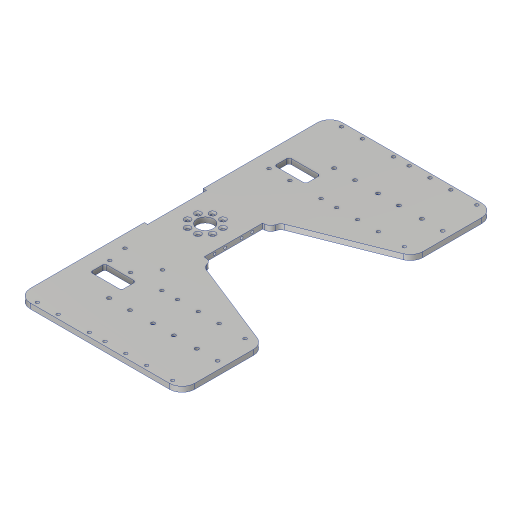
# Autodesk Inventor part: J1J2_Bottom
Saved by Autodesk Inventor 2023.2 (Build 272271000, 271)
## iProperties
Created: 2021-07-07
Part Number: J1J2_Bottom
Material: 알루미늄 6061
Document SubType Name: Modeling
Designer: user
Density: 2.7 g/cm^3
Appearance: 알루미늄 - 평지
Mass: 458.982 g
Surface Area: 798.012 cm^2
Volume: 169.993 cm^3
Author: user
Autodesk Inventor part; units mm, degrees
(part 1 of 4)
ref_plane "YZ Plane" through (0, 0, 0) normal (1, 0, 0) x (0, 1, 0)
ref_plane "XZ Plane" through (0, 0, 0) normal (0, 1, 0) x (-1, 0, 0)
ref_plane "XY Plane" through (0, 0, 0) normal (0, 0, 1) x (1, 0, 0)
sketch "스케치1" plane through (0, 0, 0) normal (0, 1, 0) x (-1, 0, 0)
  line L0 (27.1, 28) -> (-27.1, 28)
  line L1 (-27.1, 28) -> (-27.1, -28)
  line L2 (-27.1, -28) -> (27.1, -28)
  line L3 (27.1, -28) -> (27.1, 28)
  point P0 (0, 0)
  dimension "d0" = 54.2
  dimension "d1" = 56
  dimension "d2" = 27.1
  dimension "d3" = 28
  constraints: 8 end point, 2 parallel, 1 horizontal, 1 perpendicular
  measures "d0" distance of L2.end L1.end
  measures "d1" distance of L1.end L0.end
  measures "d2" distance from line of L3 point (0, 0)
  measures "d3" distance from line of L0 point (0, 0)
extrude "돌출1" add sketch "스케치1" along normal blind 5
sketch "스케치3" plane through (0, 5, 0) normal (0, 1, 0) x (1, 0, 0)
  line L0 (0, 0) -> (12.0104, 4.9749)
  line L1 (0, 0) -> (13, 0) construction
  circle A0 centre (12.0104, 4.9749) radius 1.6
  circle A1 centre (4.9749, 12.0104) radius 1.6
  circle A2 centre (-4.9749, 12.0104) radius 1.6
  circle A3 centre (-12.0104, 4.9749) radius 1.6
  circle A4 centre (-12.0104, -4.9749) radius 1.6
  circle A5 centre (-4.9749, -12.0104) radius 1.6
  circle A6 centre (4.9749, -12.0104) radius 1.6
  circle A7 centre (12.0104, -4.9749) radius 1.6
  point P0 (0, 0)
  dimension "d32" = 13
  dimension "d33" = 22.5
  dimension "d34" = 3.2
  dimension "d37" = 360
  constraints: 8 centre point, 4 end point, 1 coincident, 1 equal length, 1 horizontal, 17 other
  measures "d32" distance of L0.start L0.end
  measures "d33" angle of L1 L0
  measures "d34" diameter of A0
sketch "스케치4" plane through (0, 5, 0) normal (0, 1, 0) x (1, 0, 0)
  line L0 (27.1, 28) -> (-27.1, 28) projected
  line L1 (-27.1, -28) -> (27.1, -28) projected
  circle A0 centre (0, 0) radius 8
  line L2 (27.1, -28) -> (27.1, 28) projected
  line L3 (-27.1, 28) -> (-27.1, -28) projected
  dimension "d13" = 16
  constraints: 1 centre point, 1 coincident
  measures "d13" diameter of A0
extrude "돌출4" cut sketch "스케치4" against normal up to surface (5 mm away) contours A0
sketch "스케치5" plane through (27.1, 0, 28) normal (1, 0, 0) x (0, 0, -1)
  line L0 (0, 0) -> (56, 0) projected
  line L1 (56, 0) -> (56, 5) projected
  line L2 (0, 5) -> (56, 5) projected
  line L3 (0, 0) -> (0, 5) projected
  circle A0 centre (10, 2.5) radius 1.25
  circle A1 centre (20, 2.5) radius 1.25
  circle A2 centre (46, 2.5) radius 1.25
  circle A3 centre (36, 2.5) radius 1.25
  point P0 (28, 0)
  dimension "d16" = 2.5
  dimension "d17" = 2.5
  dimension "d18" = 2.5
  dimension "d19" = 2.5
  dimension "d20" = 2.5
  dimension "d21" = 2.5
  dimension "d22" = 2.5
  dimension "d23" = 2.5
  dimension "d24" = 10
  dimension "d25" = 20
  dimension "d26" = 20
  dimension "d27" = 10
  constraints: 4 centre point
  measures "d16" diameter of A0
  measures "d17" diameter of A1
  measures "d18" diameter of A2
  measures "d19" diameter of A3
  measures "d20" distance from line of L2 A0.centre
  measures "d21" distance from line of L2 A1.centre
  measures "d22" distance from line of L2 A2.centre
  measures "d23" distance from line of L2 A3.centre
  measures "d24" distance from line of L3 A0.centre
  measures "d25" distance from line of L3 A1.centre
  measures "d26" distance from line of L1 A3.centre
  measures "d27" distance from line of L1 A2.centre
extrude "돌출5" cut sketch "스케치5" against normal blind 8 contours A0 | A1 | A2 | A3
sketch "스케치6" plane through (-27.1, 0, -28) normal (-1, 0, 0) x (0, 0, 1)
  circle A0 centre (10, 2.5) radius 1.25 projected
  circle A1 centre (46, 2.5) radius 1.25 projected
  circle A2 centre (36, 2.5) radius 1.25 projected
  circle A3 centre (20, 2.5) radius 1.25 projected
  line L0 (56, 0) -> (0, 0) projected
  line L1 (0, 0) -> (0, 5) projected
  line L2 (56, 5) -> (0, 5) projected
  line L3 (56, 0) -> (56, 5) projected
  point P0 (28, 0)
extrude "돌출6" cut sketch "스케치6" against normal blind 8 contours A0 | A1 | A2 | A3
extrude "돌출7" cut sketch "스케치3" against normal up to surface (5 mm away)
chamfer "모따기1" distance 1.5 angle 45 8 edges at (-6.5749, 5, -12.0104) (-13.6104, 5, -4.9749) (-13.6104, 5, 4.9749) (-6.5749, 5, 12.0104) (3.3749, 5, 12.0104) (10.4104, 5, 4.9749) (10.4104, 5, -4.9749) (3.3749, 5, -12.0104)
sketch "스케치7" plane through (0, 0, 0) normal (0, -1, 0) x (1, 0, 0)
  circle A0 centre (4.9749, 12.0104) radius 1.6 projected
  circle A1 centre (12.0104, 4.9749) radius 1.6 projected
  circle A2 centre (-4.9749, 12.0104) radius 1.6 projected
  circle A3 centre (-12.0104, -4.9749) radius 1.6 projected
  circle A4 centre (4.9749, -12.0104) radius 1.6 projected
  circle A5 centre (12.0104, -4.9749) radius 1.6 projected
  circle A6 centre (-4.9749, -12.0104) radius 1.6 projected
  circle A7 centre (-12.0104, 4.9749) radius 1.6 projected
  circle A8 centre (0, 0) radius 8 projected
  line L0 (-27.1, 28) -> (27.1, 28) projected
  line L1 (-27.1, -28) -> (-27.1, 28) projected
  line L2 (27.1, -28) -> (-27.1, -28) projected
  line L3 (27.1, 28) -> (27.1, -28) projected
  line L4 (-27.1, -28) -> (-27.1, 28) projected
  line L5 (-27.1, -28) -> (156.694, -28)
  line L6 (156.694, -28) -> (156.694, -147.2716)
  line L7 (156.694, -147.2716) -> (-27.1, -147.2716)
  line L8 (-27.1, -147.2716) -> (-27.1, -28)
  line L9 (122.7787, -73) -> (-26.8765, -73)
  line L10 (-26.8765, -73) -> (-26.8765, -77)
  line L11 (-26.8765, -77) -> (122.7787, -77)
  line L12 (122.7787, -77) -> (122.7787, -73)
  line L13 (-31.8765, -68) -> (127.7787, -68)
  line L14 (127.7787, -68) -> (127.7787, -82)
  line L15 (127.7787, -82) -> (-31.8765, -82)
  line L16 (-31.8765, -82) -> (-31.8765, -68)
  point P0 (122.7787, -77)
  point P1 (-26.8765, -73)
  point P2 (-27.1, -68)
  point P3 (-27.1, -82)
  constraints: 24 end point, 4 parallel, 2 horizontal, 2 perpendicular, 4 other
extrude "돌출8" add sketch "스케치7" against normal blind 5 contours L2 L5 L6 L7 L8 L15 L14 L13
sketch "스케치9" plane through (0, 5, 0) normal (0, 1, 0) x (1, 0, 0)
  circle A0 centre (12.0104, 4.9749) radius 3.1 projected
  circle A1 centre (4.9749, -12.0104) radius 3.1 projected
  circle A2 centre (-12.0104, -4.9749) radius 3.1 projected
  circle A3 centre (-4.9749, 12.0104) radius 3.1 projected
  circle A4 centre (0, 0) radius 8 projected
  line L0 (-27.1, -28) -> (27.1, -28) projected
  line L1 (27.1, -28) -> (27.1, 28) projected
  line L2 (156.694, 28) -> (27.1, 28) projected
  line L3 (156.694, 147.2716) -> (156.694, 28) projected
  line L4 (-27.1, 147.2716) -> (156.694, 147.2716) projected
  line L5 (-27.1, 82) -> (-27.1, 147.2716) projected
  line L6 (127.7787, 82) -> (-27.1, 82) projected
  line L7 (127.7787, 68) -> (127.7787, 82) projected
  line L8 (-27.1, 68) -> (127.7787, 68) projected
  line L9 (-27.1, -28) -> (-27.1, 68) projected
  circle A5 centre (-12.0104, 4.9749) radius 3.1 projected
  circle A6 centre (-4.9749, -12.0104) radius 3.1 projected
  circle A7 centre (12.0104, -4.9749) radius 3.1 projected
  circle A8 centre (4.9749, 12.0104) radius 3.1 projected
  line L10 (57.8107, 78.5) -> (83.8107, 78.5) projected
  line L11 (127.7787, 82) -> (-27.1, 82) projected
  line L12 (83.8107, 78.5) -> (57.8107, 78.5)
  line L13 (57.8107, 78.5) -> (57.8107, 82)
  line L14 (57.8107, 82) -> (83.8107, 82)
  line L15 (83.8107, 82) -> (83.8107, 78.5)
  line L16 (70.8107, 82) -> (70.8107, 111.2)
  line L17 (70.8107, 111.2) -> (70.8107, 113.7)
  line L18 (70.8107, 96.6) -> (56.2107, 96.6)
  line L19 (56.2107, 96.6) -> (53.7107, 96.6)
  line L20 (70.8107, 96.6) -> (85.4107, 96.6)
  line L21 (85.4107, 96.6) -> (87.9107, 96.6)
  circle A9 centre (0, 0) radius 8.1
  circle A10 centre (0, 0) radius 10.1
  arc A11 (2.5, 12) -> (-2.5, 12) centre (0, 12) ccw
  arc A12 (12, -2.5) -> (12, 2.5) centre (12, 0) ccw
  arc A13 (-12, 2.5) -> (-12, -2.5) centre (-12, 0) ccw
  line L22 (2.5, 12) -> (2.5, 9.7857)
  line L23 (-2.5, 12) -> (-2.5, 9.7857)
  line L24 (-12, 2.5) -> (-9.7857, 2.5)
  line L25 (-12, -2.5) -> (-9.7857, -2.5)
  line L26 (12, 2.5) -> (9.7857, 2.5)
  line L27 (12, -2.5) -> (9.7857, -2.5)
  circle A14 centre (0, 12) radius 1.35
  circle A15 centre (12, 0) radius 1.35
  circle A16 centre (-12, 0) radius 1.35
  line L28 (58.8107, 99.1) -> (61.025, 99.1)
  line L29 (58.8107, 94.1) -> (61.025, 94.1)
  arc A17 (58.8107, 99.1) -> (58.8107, 94.1) centre (58.8107, 96.6) ccw
  circle A18 centre (58.8107, 96.6) radius 1.35
  line L30 (82.8107, 99.1) -> (80.5964, 99.1)
  circle A19 centre (82.8107, 96.6) radius 1.35
  arc A20 (82.8107, 94.1) -> (82.8107, 99.1) centre (82.8107, 96.6) ccw
  line L31 (82.8107, 94.1) -> (80.5964, 94.1)
  circle A21 centre (70.8107, 96.6) radius 8.1
  circle A22 centre (70.8107, 96.6) radius 10.1
  line L32 (68.3107, 108.6) -> (68.3107, 106.3857)
  line L33 (73.3107, 108.6) -> (73.3107, 106.3857)
  circle A23 centre (70.8107, 108.6) radius 1.35
  arc A24 (73.3107, 108.6) -> (68.3107, 108.6) centre (70.8107, 108.6) ccw
  dimension "d137" = 16.2
  dimension "d138" = 2
  dimension "d139" = 5
  dimension "d140" = 5
  dimension "d141" = 5
  dimension "d142" = 12
  dimension "d143" = 12
  dimension "d144" = 12
  dimension "d145" = 2.7
  dimension "d146" = 2.7
  dimension "d147" = 2.7
  dimension "d148" = 16.2
  dimension "d149" = 2
  dimension "d150" = 5
  dimension "d151" = 5
  dimension "d152" = 5
  dimension "d153" = 12
  dimension "d154" = 12
  dimension "d155" = 12
  dimension "d156" = 2.7
  dimension "d157" = 2.7
  dimension "d158" = 2.7
  constraints: 44 end point, 24 point on circle, 16 centre point, 11 point on line, 10 coincident, 6 tangent, 5 horizontal, 4 parallel, 4 vertical, 1 midpoint, 1 perpendicular
  measures "d137" diameter of A9
  measures "d138" radial gap between concentric circles of A9 A10
  measures "d139" diameter of A11
  measures "d140" diameter of A12
  measures "d141" diameter of A13
  measures "d142" distance of A11.centre point (0, 0)
  measures "d143" distance of A12.centre point (0, 0)
  measures "d144" distance of A13.centre point (0, 0)
  measures "d145" diameter of A14
  measures "d146" diameter of A15
  measures "d147" diameter of A16
  measures "d148" diameter of A21
  measures "d149" radial gap between concentric circles of A21 A22
  measures "d150" diameter of A24
  measures "d151" diameter of A20
  measures "d152" diameter of A17
  measures "d153" distance of A24.centre point (70.811, 96.6)
  measures "d154" distance of A20.centre point (70.811, 96.6)
  measures "d155" distance of A17.centre point (70.811, 96.6)
  measures "d156" diameter of A23
  measures "d157" diameter of A19
  measures "d158" diameter of A18
extrude "돌출9" cut sketch "스케치9" against normal blind 5 contours A18 L18 | L18 A18 | A19 L20 | L20 A19 | A23 L16 | L16 A23
sketch "스케치13" plane through (0, 5, 0) normal (0, 1, 0) x (1, 0, 0)
  line L0 (127.7787, 82) -> (-27.1, 82) projected
  line L1 (127.7787, 68) -> (127.7787, 82) projected
  line L2 (-27.1, 68) -> (127.7787, 68) projected
  line L3 (-27.1, -28) -> (-27.1, 68) projected
  line L4 (-27.1, -28) -> (27.1, -28) projected
  line L5 (27.1, -28) -> (27.1, 28) projected
  line L6 (156.694, 28) -> (27.1, 28) projected
  line L7 (156.694, 147.2716) -> (156.694, 28) projected
  line L8 (-27.1, 147.2716) -> (156.694, 147.2716) projected
  line L9 (-27.1, 82) -> (-27.1, 147.2716) projected
  circle A0 centre (12.0104, 4.9749) radius 3.1 projected
  circle A1 centre (4.9749, -12.0104) radius 3.1 projected
  circle A2 centre (-12.0104, -4.9749) radius 3.1 projected
  circle A3 centre (-4.9749, 12.0104) radius 3.1 projected
  circle A4 centre (0, 0) radius 8 projected
  circle A5 centre (-12.0104, 4.9749) radius 3.1 projected
  circle A6 centre (-4.9749, -12.0104) radius 3.1 projected
  circle A7 centre (12.0104, -4.9749) radius 3.1 projected
  circle A8 centre (4.9749, 12.0104) radius 3.1 projected
  line L10 (27.1, -28) -> (27.1, 28) projected
  line L11 (-27.1, 68) -> (127.7787, 68) projected
  line L12 (27.1, 28) -> (127.7787, 68)
  line L13 (-27.1, 82) -> (-27.1, 147.2716) projected
  line L14 (127.7787, 68) -> (-27.1, 68)
  line L15 (-27.1, 68) -> (-27.1, 147.2716)
  line L16 (-27.1, 147.2716) -> (127.7787, 147.2716)
  line L17 (127.7787, 147.2716) -> (127.7787, 68)
  line L18 (-27.1, 147.2716) -> (156.694, 147.2716) projected
  line L19 (-27.1, 147.2716) -> (127.7787, 147.2716)
  line L20 (127.7787, 147.2716) -> (127.7787, 117.4659)
  line L21 (127.7787, 117.4659) -> (-27.1, 117.4659)
  line L22 (-27.1, 117.4659) -> (-27.1, 147.2716)
  constraints: 18 end point, 4 parallel, 2 horizontal, 2 perpendicular, 1 point on line
extrude "돌출13" cut sketch "스케치13" against normal blind 500 contours L17 L8 L7 L6 L12 L1 | L21 L9 L8 L17
sketch "스케치14" plane through (0, 0, 0) normal (0, -1, 0) x (1, 0, 0)
  line L0 (-27.1, -117.4659) -> (127.7787, -117.4659) projected
  line L1 (127.7787, -117.4659) -> (127.7787, -82) projected
  line L2 (127.7787, -82) -> (-27.1, -82) projected
  line L3 (-27.1, -82) -> (-27.1, -117.4659) projected
  line L4 (127.7787, -68) -> (27.1, -28) projected
  line L5 (27.1, 28) -> (27.1, -28) projected
  line L6 (-27.1, 28) -> (27.1, 28) projected
  line L7 (-27.1, 28) -> (-27.1, -68) projected
  line L8 (-27.1, -68) -> (127.7787, -68) projected
  circle A0 centre (4.9749, 12.0104) radius 1.6 projected
  circle A1 centre (12.0104, 4.9749) radius 1.6 projected
  circle A2 centre (-4.9749, 12.0104) radius 1.6 projected
  circle A3 centre (-12.0104, -4.9749) radius 1.6 projected
  circle A4 centre (4.9749, -12.0104) radius 1.6 projected
  circle A5 centre (12.0104, -4.9749) radius 1.6 projected
  circle A6 centre (-4.9749, -12.0104) radius 1.6 projected
  circle A7 centre (-12.0104, 4.9749) radius 1.6 projected
  circle A8 centre (0, 0) radius 8 projected
  line L9 (92.0011, -83.5) -> (92.0011, -78.5) projected
  line L10 (49.6203, -83.5) -> (49.6203, -78.5) projected
  line L11 (-27.1, -68) -> (127.7787, -68) projected
  line L12 (127.7787, -82) -> (-27.1, -82) projected
  line L13 (127.7787, -68) -> (92.0011, -68)
  line L14 (92.0011, -68) -> (92.0011, -82)
  line L15 (92.0011, -82) -> (127.7787, -82)
  line L16 (127.7787, -82) -> (127.7787, -68)
  line L17 (49.6203, -82) -> (-27.1, -82)
  line L18 (-27.1, -82) -> (-27.1, -68)
  line L19 (-27.1, -68) -> (49.6203, -68)
  line L20 (49.6203, -68) -> (49.6203, -82)
  point P0 (92.0011, -82)
  constraints: 16 end point, 4 parallel, 4 point on line, 2 horizontal, 2 perpendicular
extrude "돌출14" add sketch "스케치14" against normal blind 5 contours L18 L8 L20 L10 L2 | L2 L9 L14 L8 L16
sketch "스케치15" plane through (0, 5, 0) normal (0, 1, 0) x (1, 0, 0)
  line L0 (92.0011, 82) -> (49.6203, 82) projected
  line L1 (92.0011, 68) -> (92.0011, 82) projected
  line L2 (49.6203, 68) -> (92.0011, 68) projected
  line L3 (49.6203, 82) -> (49.6203, 68) projected
  circle A0 centre (4.9749, 12.0104) radius 3.1 projected
  circle A1 centre (12.0104, -4.9749) radius 3.1 projected
  circle A2 centre (-4.9749, -12.0104) radius 3.1 projected
  circle A3 centre (-12.0104, 4.9749) radius 3.1 projected
  circle A4 centre (0, 0) radius 8 projected
  circle A5 centre (-4.9749, 12.0104) radius 3.1 projected
  circle A6 centre (-12.0104, -4.9749) radius 3.1 projected
  circle A7 centre (4.9749, -12.0104) radius 3.1 projected
  circle A8 centre (12.0104, 4.9749) radius 3.1 projected
  line L4 (-27.1, -28) -> (-27.1, 117.4659) projected
  line L5 (-27.1, -28) -> (27.1, -28) projected
  line L6 (27.1, -28) -> (27.1, 28) projected
  line L7 (27.1, 28) -> (127.7787, 68) projected
  line L8 (127.7787, 117.4659) -> (127.7787, 68) projected
  line L9 (127.7787, 117.4659) -> (-27.1, 117.4659) projected
  line L10 (127.7787, 117.4659) -> (-27.1, 117.4659) projected
  line L11 (-27.1, 117.4659) -> (15.1104, 117.4659)
  line L12 (15.1104, 117.4659) -> (15.1104, 82)
  line L13 (15.1104, 82) -> (-27.1, 82)
  line L14 (-27.1, 82) -> (-27.1, 117.4659)
  point P0 (15.1104, 117.4659)
  constraints: 8 end point, 2 parallel, 1 horizontal, 1 perpendicular
extrude "돌출15" cut sketch "스케치15" against normal blind 5 contours L4 L9 L12 L13
chamfer "모따기3" distance 2 angle 45 1 edges at (127.7787, 2.5, -68)
sketch "스케치16" plane through (0, 0, 0) normal (0, -1, 0) x (1, 0, 0)
  line L0 (49.6203, -82) -> (49.6203, -68) projected
  line L1 (49.6203, -68) -> (92.0011, -68) projected
  line L2 (92.0011, -68) -> (92.0011, -82) projected
  line L3 (92.0011, -82) -> (49.6203, -82) projected
  circle A0 centre (4.9749, 12.0104) radius 1.6 projected
  circle A1 centre (12.0104, 4.9749) radius 1.6 projected
  circle A2 centre (-4.9749, 12.0104) radius 1.6 projected
  circle A3 centre (-12.0104, -4.9749) radius 1.6 projected
  circle A4 centre (4.9749, -12.0104) radius 1.6 projected
  circle A5 centre (12.0104, -4.9749) radius 1.6 projected
  circle A6 centre (-4.9749, -12.0104) radius 1.6 projected
  circle A7 centre (-12.0104, 4.9749) radius 1.6 projected
  circle A8 centre (0, 0) radius 8 projected
  line L4 (125.92, -67.2615) -> (127.7787, -70) projected
  line L5 (125.92, -67.2615) -> (27.1, -28) projected
  line L6 (27.1, 28) -> (27.1, -28) projected
  line L7 (-27.1, 28) -> (27.1, 28) projected
  line L8 (-27.1, 28) -> (-27.1, -82) projected
  line L9 (-27.1, -82) -> (15.1104, -82) projected
  line L10 (15.1104, -82) -> (15.1104, -117.4659) projected
  line L11 (15.1104, -117.4659) -> (127.7787, -117.4659) projected
  line L12 (127.7787, -117.4659) -> (127.7787, -70) projected
  circle A9 centre (31.6, -60) radius 1 projected
  circle A10 centre (89.8107, -60) radius 1 projected
  line L13 (-24.9, -58) -> (97.8107, -58) projected
  line L14 (-24.9, -58) -> (-24.9, -62) projected
  line L15 (97.8107, -62) -> (-24.9, -62) projected
  line L16 (97.8107, -58) -> (97.8107, -62) projected
  line L17 (0, 4) -> (122.7107, 4)
  line L18 (0, 4) -> (0, 0)
  line L19 (122.7107, 0) -> (0, 0)
  line L20 (122.7107, 4) -> (122.7107, 0)
  line L21 (122.7107, 4) -> (122.7107, 0)
  line L22 (122.7107, 2) -> (114.7107, 2)
  circle A11 centre (114.7107, 2) radius 1.25
  line L23 (50.5, 0) -> (47.5, 0)
  line L24 (50.5, 4) -> (47.5, 4)
  circle A12 centre (94.7107, 2) radius 1.25
  circle A13 centre (74.7107, 2) radius 1.25
  circle A14 centre (14, 2) radius 1.25
  circle A15 centre (34, 2) radius 1.25
  line L25 (-2, 4) -> (-2, 0)
  circle A16 centre (64, 2) radius 1.25
  circle A17 centre (-10.9, -60) radius 1.6
  circle A18 centre (9.1, -60) radius 1.6
  circle A19 centre (39.1, -60) radius 1.6
  circle A20 centre (49.8107, -60) radius 1.6
  circle A21 centre (69.8107, -60) radius 1.6
  circle A22 centre (89.8107, -60) radius 1.6
  point P0 (-2, 2)
  point P1 (-24.9, -60)
  point P2 (97.8107, -60)
  dimension "d111" = 8
  dimension "d112" = 2.5
  dimension "d113" = 2.5
  dimension "d114" = 20
  dimension "d115" = 2.5
  dimension "d116" = 20
  dimension "d117" = 2.5
  dimension "d118" = 2.5
  dimension "d119" = 20
  dimension "d120" = 16
  dimension "d121" = 2.5
  dimension "d122" = 30
  dimension "d123" = 3.2
  dimension "d124" = 3.2
  dimension "d125" = 20
  dimension "d127" = 3.2
  dimension "d128" = 3.2
  dimension "d129" = 3.2
  dimension "d130" = 30
  dimension "d131" = 20
  dimension "d132" = 3.2
  dimension "d133" = 20
  dimension "d134" = 8
  dimension "d136" = 14
  constraints: 18 end point, 12 centre point, 4 midpoint, 1 coincident, 1 horizontal
  measures "d111" distance of L22.start L22.end
  measures "d112" diameter of A11
  measures "d113" diameter of A12
  measures "d114" distance of A12.centre L22.end
  measures "d115" diameter of A13
  measures "d116" distance of A13.centre A12.centre
  measures "d117" diameter of A14
  measures "d118" diameter of A15
  measures "d119" distance of A14.centre A15.centre
  measures "d120" distance of point (-2, 2) A14.centre
  measures "d121" diameter of A16
  measures "d122" distance of A15.centre A16.centre
  measures "d123" diameter of A17
  measures "d124" diameter of A18
  measures "d125" distance of A17.centre A18.centre
  measures "d127" diameter of A19
  measures "d128" diameter of A20
  measures "d129" diameter of A21
  measures "d130" distance of A19.centre A18.centre
  measures "d131" distance of A21.centre A20.centre
  measures "d132" diameter of A22
  measures "d133" distance of A21.centre A22.centre
  measures "d134" distance of point (97.811, -60) A22.centre
  measures "d136" distance of point (-24.9, -60) A17.centre
extrude "돌출16" cut sketch "스케치16" against normal blind 10 contours A10 | A17 | A18 | A19 | A20 | A21 | A22
fillet "모깎기2" radius 2 4 edges at (49.6203, 2.5, -82) (49.6203, 2.5, -68) (92.0011, 2.5, -68) (92.0011, 2.5, -82)
sketch "스케치17" plane through (0, 5, 0) normal (0, 1, 0) x (1, 0, 0)
  line L0 (127.7787, 70) -> (125.92, 67.2615) projected
  line L1 (127.7787, 117.4659) -> (127.7787, 70) projected
  line L2 (127.7787, 117.4659) -> (15.1104, 117.4659) projected
  line L3 (15.1104, 117.4659) -> (15.1104, 82) projected
  line L4 (15.1104, 82) -> (-27.1, 82) projected
  line L5 (-27.1, -28) -> (-27.1, 82) projected
  line L6 (-27.1, -28) -> (27.1, -28) projected
  line L7 (27.1, -28) -> (27.1, 28) projected
  line L8 (27.1, 28) -> (125.92, 67.2615) projected
  line L9 (90.0011, 82) -> (51.6203, 82) projected
  arc A0 (92.0011, 80) -> (90.0011, 82) centre (90.0011, 80) ccw projected
  line L10 (92.0011, 70) -> (92.0011, 80) projected
  arc A1 (90.0011, 68) -> (92.0011, 70) centre (90.0011, 70) ccw projected
  line L11 (51.6203, 68) -> (90.0011, 68) projected
  arc A2 (49.6203, 70) -> (51.6203, 68) centre (51.6203, 70) ccw projected
  line L12 (49.6203, 80) -> (49.6203, 70) projected
  arc A3 (51.6203, 82) -> (49.6203, 80) centre (51.6203, 80) ccw projected
  circle A4 centre (4.9749, 12.0104) radius 3.1 projected
  circle A5 centre (12.0104, -4.9749) radius 3.1 projected
  circle A6 centre (-4.9749, -12.0104) radius 3.1 projected
  circle A7 centre (-12.0104, 4.9749) radius 3.1 projected
  circle A8 centre (0, 0) radius 8 projected
  circle A9 centre (-4.9749, 12.0104) radius 3.1 projected
  circle A10 centre (-12.0104, -4.9749) radius 3.1 projected
  circle A11 centre (4.9749, -12.0104) radius 3.1 projected
  circle A12 centre (12.0104, 4.9749) radius 3.1 projected
  line L13 (27.1, 28) -> (125.92, 67.2615) projected
  line L14 (27.1, 28) -> (27.1, 30)
  line L15 (27.1, 30) -> (127.7787, 70)
  line L16 (-27.1, 80) -> (-27.1, 117.4659)
  line L17 (125.7787, 117.4659) -> (17.1104, 117.4659) projected
  line L18 (-27.1, 117.4659) -> (17.1104, 117.4659)
  dimension "d98" = 2
  constraints: 8 end point, 2 vertical, 1 collinear
  measures "d98" distance of L7.end L14.end
extrude "돌출17" cut sketch "스케치17" against normal blind 10 contours L0 L8 L14 L15
extrude "돌출18" add sketch "스케치17" against normal up to surface (5 mm away) contours L3 L4 L16 L18
sketch "스케치18" plane through (0, 5, 0) normal (0, 1, 0) x (1, 0, 0)
  circle A0 centre (12.0104, 4.9749) radius 3.1 projected
  circle A1 centre (4.9749, -12.0104) radius 3.1 projected
  circle A2 centre (-12.0104, -4.9749) radius 3.1 projected
  circle A3 centre (-4.9749, 12.0104) radius 3.1 projected
  circle A4 centre (0, 0) radius 8 projected
  circle A5 centre (-12.0104, 4.9749) radius 3.1 projected
  circle A6 centre (-4.9749, -12.0104) radius 3.1 projected
  circle A7 centre (12.0104, -4.9749) radius 3.1 projected
  circle A8 centre (4.9749, 12.0104) radius 3.1 projected
  line L0 (90.0011, 82) -> (51.6203, 82) projected
  arc A9 (92.0011, 80) -> (90.0011, 82) centre (90.0011, 80) ccw projected
  line L1 (92.0011, 70) -> (92.0011, 80) projected
  arc A10 (90.0011, 68) -> (92.0011, 70) centre (90.0011, 70) ccw projected
  line L2 (51.6203, 68) -> (90.0011, 68) projected
  arc A11 (49.6203, 70) -> (51.6203, 68) centre (51.6203, 70) ccw projected
  line L3 (49.6203, 80) -> (49.6203, 70) projected
  arc A12 (51.6203, 82) -> (49.6203, 80) centre (51.6203, 80) ccw projected
  line L4 (27.1, -28) -> (27.1, 30) projected
  line L5 (27.1, 30) -> (127.7787, 70) projected
  line L6 (127.7787, 117.4659) -> (127.7787, 70) projected
  line L7 (127.7787, 117.4659) -> (-27.1, 117.4659) projected
  line L8 (-27.1, 117.4659) -> (-27.1, -28) projected
  line L9 (-27.1, -28) -> (27.1, -28) projected
  line L10 (92.0011, 70) -> (92.0011, 80) projected
  line L11 (92.0011, 75) -> (-27.1, 75)
  line L12 (-27.1, 117.4659) -> (-27.1, -28) projected
  line L13 (-15, 68) -> (15, 68)
  line L14 (15, 68) -> (15, 82)
  line L15 (15, 82) -> (-15, 82)
  line L16 (-15, 82) -> (-15, 68)
  line L17 (-15, 68) -> (15, 82) construction
  line L18 (15, 68) -> (-15, 82) construction
  point P0 (0, 75)
  dimension "d103" = 30
  constraints: 14 end point, 3 midpoint, 3 point on line, 2 parallel, 2 perpendicular, 1 horizontal
  measures "d103" distance of L15.end L14.end
extrude "돌출19" cut sketch "스케치18" against normal blind 10 contours L14 L13 L16 L11 | L11 L16 L15 L14
sketch "스케치19" plane through (0, 5, 0) normal (0, 1, 0) x (1, 0, 0)
  line L0 (-15, 82) -> (15, 82) projected
  line L1 (15, 82) -> (15, 68) projected
  line L2 (15, 68) -> (-15, 68) projected
  line L3 (-15, 68) -> (-15, 82) projected
  circle A0 centre (12.0104, 4.9749) radius 3.1 projected
  circle A1 centre (4.9749, -12.0104) radius 3.1 projected
  circle A2 centre (-12.0104, -4.9749) radius 3.1 projected
  circle A3 centre (-4.9749, 12.0104) radius 3.1 projected
  circle A4 centre (0, 0) radius 8 projected
  circle A5 centre (-12.0104, 4.9749) radius 3.1 projected
  circle A6 centre (-4.9749, -12.0104) radius 3.1 projected
  circle A7 centre (12.0104, -4.9749) radius 3.1 projected
  circle A8 centre (4.9749, 12.0104) radius 3.1 projected
  line L4 (90.0011, 82) -> (51.6203, 82) projected
  arc A9 (92.0011, 80) -> (90.0011, 82) centre (90.0011, 80) ccw projected
  line L5 (92.0011, 70) -> (92.0011, 80) projected
  arc A10 (90.0011, 68) -> (92.0011, 70) centre (90.0011, 70) ccw projected
  line L6 (51.6203, 68) -> (90.0011, 68) projected
  arc A11 (49.6203, 70) -> (51.6203, 68) centre (51.6203, 70) ccw projected
  line L7 (49.6203, 80) -> (49.6203, 70) projected
  arc A12 (51.6203, 82) -> (49.6203, 80) centre (51.6203, 80) ccw projected
  line L8 (27.1, -28) -> (27.1, 30) projected
  line L9 (27.1, 30) -> (127.7787, 70) projected
  line L10 (127.7787, 117.4659) -> (127.7787, 70) projected
  line L11 (127.7787, 117.4659) -> (-27.1, 117.4659) projected
  line L12 (-27.1, 117.4659) -> (-27.1, -28) projected
  line L13 (-27.1, -28) -> (27.1, -28) projected
  line L14 (-27.1, -28) -> (-27.1, 117.4659) projected
  line L15 (-27.1, 97.4659) -> (12.9, 117.4659)
  line L16 (-27.1, 117.4659) -> (125.7787, 117.4659) projected
  dimension "d106" = 20
  dimension "d107" = 40
  constraints: 2 end point, 2 point on line
  measures "d106" distance from line of L15.start L16
  measures "d107" distance from line of L12 L15.end
extrude "돌출20" cut sketch "스케치19" against normal blind 10 contours L12 L11 L15
fillet "모깎기3" radius 2 9 edges at (15, 2.5, -68) (15, 2.5, -82) (-15, 2.5, -68) (-15, 2.5, -82) (-27.1, 2.5, -97.4659) (12.9, 2.5, -117.4659) (127.7787, 2.5, -117.4659) (127.7787, 2.5, -70) (27.1, 2.5, -30)
sketch "스케치20" plane through (0, 5, 0) normal (0, 1, 0) x (1, 0, 0)
  arc A0 (126.5171, 69.4988) -> (127.7787, 71.3575) centre (125.7787, 71.3575) ccw projected
  line L0 (127.7787, 115.4659) -> (127.7787, 71.3575) projected
  arc A1 (127.7787, 115.4659) -> (125.7787, 117.4659) centre (125.7787, 115.4659) ccw projected
  line L1 (125.7787, 117.4659) -> (13.3721, 117.4659) projected
  arc A2 (13.3721, 117.4659) -> (12.4777, 117.2547) centre (13.3721, 115.4659) ccw projected
  line L2 (12.4777, 117.2547) -> (-25.9944, 98.0187) projected
  arc A3 (-25.9944, 98.0187) -> (-27.1, 96.2298) centre (-25.1, 96.2298) ccw projected
  line L3 (-27.1, 96.2298) -> (-27.1, -28) projected
  line L4 (-27.1, -28) -> (27.1, -28) projected
  line L5 (27.1, -28) -> (27.1, 28.6425) projected
  arc A4 (28.3615, 30.5012) -> (27.1, 28.6425) centre (29.1, 28.6425) ccw projected
  line L6 (28.3615, 30.5012) -> (126.5171, 69.4988) projected
  line L7 (15, 80) -> (15, 70) projected
  arc A5 (13, 68) -> (15, 70) centre (13, 70) ccw projected
  line L8 (13, 68) -> (-13, 68) projected
  arc A6 (-15, 70) -> (-13, 68) centre (-13, 70) ccw projected
  line L9 (-15, 70) -> (-15, 80) projected
  arc A7 (-13, 82) -> (-15, 80) centre (-13, 80) ccw projected
  line L10 (-13, 82) -> (13, 82) projected
  arc A8 (15, 80) -> (13, 82) centre (13, 80) ccw projected
  arc A9 (92.0011, 80) -> (90.0011, 82) centre (90.0011, 80) ccw projected
  line L11 (92.0011, 70) -> (92.0011, 80) projected
  arc A10 (90.0011, 68) -> (92.0011, 70) centre (90.0011, 70) ccw projected
  line L12 (51.6203, 68) -> (90.0011, 68) projected
  arc A11 (49.6203, 70) -> (51.6203, 68) centre (51.6203, 70) ccw projected
  line L13 (49.6203, 80) -> (49.6203, 70) projected
  arc A12 (51.6203, 82) -> (49.6203, 80) centre (51.6203, 80) ccw projected
  line L14 (90.0011, 82) -> (51.6203, 82) projected
  circle A13 centre (82.8107, 96.6) radius 1.35 projected
  circle A14 centre (58.8107, 96.6) radius 1.35 projected
  circle A15 centre (70.8107, 108.6) radius 1.35 projected
  circle A16 centre (4.9749, 12.0104) radius 3.1 projected
  circle A17 centre (12.0104, -4.9749) radius 3.1 projected
  circle A18 centre (-4.9749, -12.0104) radius 3.1 projected
  circle A19 centre (-12.0104, 4.9749) radius 3.1 projected
  circle A20 centre (0, 0) radius 8 projected
  circle A21 centre (-4.9749, 12.0104) radius 3.1 projected
  circle A22 centre (-12.0104, -4.9749) radius 3.1 projected
  circle A23 centre (4.9749, -12.0104) radius 3.1 projected
  circle A24 centre (12.0104, 4.9749) radius 3.1 projected
  circle A25 centre (89.8107, 60) radius 1.6 projected
  circle A26 centre (9.1, 60) radius 1.6 projected
  circle A27 centre (39.1, 60) radius 1.6 projected
  circle A28 centre (69.8107, 60) radius 1.6 projected
  circle A29 centre (-10.9, 60) radius 1.6 projected
  circle A30 centre (49.8107, 60) radius 1.6 projected
  line L15 (127.7787, 115.4659) -> (127.7787, 117.4659)
  line L16 (127.7787, 117.4659) -> (127.7787, 133.9669)
  line L17 (127.7787, 133.9669) -> (13, 133.9669)
  line L18 (13, 133.9669) -> (-27.1, 113.9169)
  line L19 (-27.1, -28) -> (-27.1, 96.2298) projected
  line L20 (-27.1, 96.2298) -> (-27.1, 113.9169)
  dimension "d159" = 16.501
  constraints: 10 end point, 2 vertical, 1 collinear, 1 parallel, 1 perpendicular, 1 tangent
  measures "d159" distance of L15.end L16.end
extrude "돌출21" add sketch "스케치20" against normal blind 5 contours A1 L1 A2 L2 A3 L20 L18 L17 L16 L15
sketch "스케치21" plane through (0, 5, 0) normal (0, 1, 0) x (1, 0, 0)
  arc A0 (126.5171, 69.4988) -> (127.7787, 71.3575) centre (125.7787, 71.3575) ccw projected
  line L0 (127.7787, 133.9669) -> (127.7787, 71.3575) projected
  line L1 (127.7787, 133.9669) -> (13, 133.9669) projected
  line L2 (13, 133.9669) -> (-27.1, 113.9169) projected
  line L3 (-27.1, 113.9169) -> (-27.1, -28) projected
  line L4 (-27.1, -28) -> (27.1, -28) projected
  line L5 (27.1, -28) -> (27.1, 28.6425) projected
  arc A1 (28.3615, 30.5012) -> (27.1, 28.6425) centre (29.1, 28.6425) ccw projected
  line L6 (28.3615, 30.5012) -> (126.5171, 69.4988) projected
  line L7 (15, 80) -> (15, 70) projected
  arc A2 (13, 68) -> (15, 70) centre (13, 70) ccw projected
  line L8 (13, 68) -> (-13, 68) projected
  arc A3 (-15, 70) -> (-13, 68) centre (-13, 70) ccw projected
  line L9 (-15, 70) -> (-15, 80) projected
  arc A4 (-13, 82) -> (-15, 80) centre (-13, 80) ccw projected
  line L10 (-13, 82) -> (13, 82) projected
  arc A5 (15, 80) -> (13, 82) centre (13, 80) ccw projected
  arc A6 (92.0011, 80) -> (90.0011, 82) centre (90.0011, 80) ccw projected
  line L11 (92.0011, 70) -> (92.0011, 80) projected
  arc A7 (90.0011, 68) -> (92.0011, 70) centre (90.0011, 70) ccw projected
  line L12 (51.6203, 68) -> (90.0011, 68) projected
  arc A8 (49.6203, 70) -> (51.6203, 68) centre (51.6203, 70) ccw projected
  line L13 (49.6203, 80) -> (49.6203, 70) projected
  arc A9 (51.6203, 82) -> (49.6203, 80) centre (51.6203, 80) ccw projected
  line L14 (90.0011, 82) -> (51.6203, 82) projected
  circle A10 centre (82.8107, 96.6) radius 1.35 projected
  circle A11 centre (58.8107, 96.6) radius 1.35 projected
  circle A12 centre (70.8107, 108.6) radius 1.35 projected
  circle A13 centre (4.9749, 12.0104) radius 3.1 projected
  circle A14 centre (12.0104, -4.9749) radius 3.1 projected
  circle A15 centre (-4.9749, -12.0104) radius 3.1 projected
  circle A16 centre (-12.0104, 4.9749) radius 3.1 projected
  circle A17 centre (0, 0) radius 8 projected
  circle A18 centre (-4.9749, 12.0104) radius 3.1 projected
  circle A19 centre (-12.0104, -4.9749) radius 3.1 projected
  circle A20 centre (4.9749, -12.0104) radius 3.1 projected
  circle A21 centre (12.0104, 4.9749) radius 3.1 projected
  circle A22 centre (89.8107, 60) radius 1.6 projected
  circle A23 centre (9.1, 60) radius 1.6 projected
  circle A24 centre (39.1, 60) radius 1.6 projected
  circle A25 centre (69.8107, 60) radius 1.6 projected
  circle A26 centre (-10.9, 60) radius 1.6 projected
  circle A27 centre (49.8107, 60) radius 1.6 projected
  arc A28 (126.5171, 85.9998) -> (127.7787, 87.8585) centre (125.7787, 87.8585) ccw
  line L15 (127.7787, 150.4679) -> (127.7787, 87.8585)
  line L16 (127.7787, 150.4679) -> (13, 150.4679)
  line L17 (13, 150.4679) -> (-27.1, 130.4179)
  line L18 (-27.1, 130.4179) -> (-27.1, -11.499)
  line L19 (-27.1, -11.499) -> (27.1, -11.499)
  line L20 (27.1, -11.499) -> (27.1, 45.1435)
  arc A29 (28.3615, 47.0022) -> (27.1, 45.1435) centre (29.1, 45.1435) ccw
  line L21 (28.3615, 47.0022) -> (126.5171, 85.9998)
  line L22 (15, 96.501) -> (15, 86.501)
  arc A30 (13, 84.501) -> (15, 86.501) centre (13, 86.501) ccw
  line L23 (13, 84.501) -> (-13, 84.501)
  arc A31 (-15, 86.501) -> (-13, 84.501) centre (-13, 86.501) ccw
  line L24 (-15, 86.501) -> (-15, 96.501)
  arc A32 (-13, 98.501) -> (-15, 96.501) centre (-13, 96.501) ccw
  line L25 (-13, 98.501) -> (13, 98.501)
  arc A33 (15, 96.501) -> (13, 98.501) centre (13, 96.501) ccw
  arc A34 (92.0011, 96.501) -> (90.0011, 98.501) centre (90.0011, 96.501) ccw
  line L26 (92.0011, 86.501) -> (92.0011, 96.501)
  arc A35 (90.0011, 84.501) -> (92.0011, 86.501) centre (90.0011, 86.501) ccw
  line L27 (51.6203, 84.501) -> (90.0011, 84.501)
  arc A36 (49.6203, 86.501) -> (51.6203, 84.501) centre (51.6203, 86.501) ccw
  line L28 (49.6203, 96.501) -> (49.6203, 86.501)
  arc A37 (51.6203, 98.501) -> (49.6203, 96.501) centre (51.6203, 96.501) ccw
  line L29 (90.0011, 98.501) -> (51.6203, 98.501)
  circle A38 centre (82.8107, 113.101) radius 1.35
  circle A39 centre (58.8107, 113.101) radius 1.35
  circle A40 centre (70.8107, 125.101) radius 1.35
  circle A41 centre (112.9107, 103.101) radius 1.75
  circle A42 centre (28.7107, 103.101) radius 1.75
  circle A43 centre (112.9107, 123.101) radius 1.75
  circle A44 centre (28.7107, 123.101) radius 1.75
  circle A45 centre (4.9749, 28.5114) radius 3.1
  circle A46 centre (12.0104, 11.5261) radius 3.1
  circle A47 centre (-4.9749, 4.4906) radius 3.1
  circle A48 centre (-12.0104, 21.4759) radius 3.1
  circle A49 centre (0, 16.501) radius 8
  circle A50 centre (-4.9749, 28.5114) radius 3.1
  circle A51 centre (-12.0104, 11.5261) radius 3.1
  circle A52 centre (4.9749, 4.4906) radius 3.1
  circle A53 centre (12.0104, 21.4759) radius 3.1
  circle A54 centre (89.8107, 76.501) radius 1.6
  circle A55 centre (9.1, 76.501) radius 1.6
  circle A56 centre (39.1, 76.501) radius 1.6
  circle A57 centre (69.8107, 76.501) radius 1.6
  circle A58 centre (-10.9, 76.501) radius 1.6
  circle A59 centre (49.8107, 76.501) radius 1.6
  circle A60 centre (-10.9, 60) radius 1.6 projected
  line L30 (-10.9, 60) -> (-10.9, 76.501)
  point P0 (0, 16.501)
  point P1 (81.2123, 68)
  point P2 (92.0011, 72.2864)
  point P3 (127.7787, 87.8585)
  dimension "d162" = 16.501
  constraints: 32 centre point, 32 end point, 20 point on circle, 1 vertical
  measures "d162" distance of L30.start L30.end
extrude "돌출22" add sketch "스케치21" against normal blind 5 contours L21 L12 A8 L13 A59 A9 L14 A6 L11 | L13 A59 | L7 A2 L8 A3 L9 A4 L10 A5 | A10 | A11 | A12 | A23 | A24 | A26 | A27 picked at (50.6624, 76.7486)
extrude "돌출23" cut sketch "스케치21" against normal blind 5 contours L6 A1 L20 A29 L21 L12 A7 L11 A28 L0 A0 | A59 L13 | L13 A59 | A10 | A11 | L22 A30 L23 A31 L24 A32 L25 A33 | L26 A35 L27 A36 L28 A37 L29 A34 | A38 | A39 | A40 | A41 | A42 | A43 | A44 | A56
sketch "스케치22" plane through (0, 5, 0) normal (0, 1, 0) x (1, 0, 0)
  line L0 (28.3615, 47.0022) -> (126.5171, 85.9998) projected
  arc A0 (126.5171, 85.9998) -> (127.7787, 87.8585) centre (125.7787, 87.8585) ccw projected
  line L1 (127.7787, 133.9669) -> (127.7787, 87.8585) projected
  line L2 (127.7787, 133.9669) -> (13, 133.9669) projected
  line L3 (13, 133.9669) -> (-27.1, 113.9169) projected
  line L4 (-27.1, 113.9169) -> (-27.1, -28) projected
  line L5 (-27.1, -28) -> (27.1, -28) projected
  line L6 (27.1, -28) -> (27.1, 45.1435) projected
  arc A1 (28.3615, 47.0022) -> (27.1, 45.1435) centre (29.1, 45.1435) ccw projected
  arc A2 (15, 96.501) -> (13, 98.501) centre (13, 96.501) ccw projected
  line L7 (15, 96.501) -> (15, 86.501) projected
  arc A3 (13, 84.501) -> (15, 86.501) centre (13, 86.501) ccw projected
  line L8 (13, 84.501) -> (-13, 84.501) projected
  arc A4 (-15, 86.501) -> (-13, 84.501) centre (-13, 86.501) ccw projected
  line L9 (-15, 86.501) -> (-15, 96.501) projected
  arc A5 (-13, 98.501) -> (-15, 96.501) centre (-13, 96.501) ccw projected
  line L10 (-13, 98.501) -> (13, 98.501) projected
  circle A6 centre (58.8107, 113.101) radius 1.35 projected
  circle A7 centre (112.9107, 103.101) radius 1.75 projected
  circle A8 centre (28.7107, 123.101) radius 1.75 projected
  circle A9 centre (82.8107, 113.101) radius 1.35 projected
  line L11 (51.6203, 98.501) -> (90.0011, 98.501) projected
  arc A10 (92.0011, 96.501) -> (90.0011, 98.501) centre (90.0011, 96.501) ccw projected
  line L12 (92.0011, 96.501) -> (92.0011, 86.501) projected
  arc A11 (90.0011, 84.501) -> (92.0011, 86.501) centre (90.0011, 86.501) ccw projected
  line L13 (90.0011, 84.501) -> (51.6203, 84.501) projected
  arc A12 (49.6203, 86.501) -> (51.6203, 84.501) centre (51.6203, 86.501) ccw projected
  line L14 (49.6203, 86.501) -> (49.6203, 96.501) projected
  arc A13 (51.6203, 98.501) -> (49.6203, 96.501) centre (51.6203, 96.501) ccw projected
  circle A14 centre (39.1, 76.501) radius 1.6 projected
  circle A15 centre (70.8107, 125.101) radius 1.35 projected
  circle A16 centre (112.9107, 123.101) radius 1.75 projected
  circle A17 centre (28.7107, 103.101) radius 1.75 projected
  circle A18 centre (49.8107, 76.501) radius 1.6 projected
  circle A19 centre (9.1, 76.501) radius 1.6 projected
  circle A20 centre (-10.9, 76.501) radius 1.6 projected
  circle A21 centre (69.8107, 76.501) radius 1.6 projected
  circle A22 centre (89.8107, 76.501) radius 1.6 projected
  circle A23 centre (12.0104, 4.9749) radius 3.1 projected
  circle A24 centre (4.9749, -12.0104) radius 3.1 projected
  circle A25 centre (-12.0104, -4.9749) radius 3.1 projected
  circle A26 centre (-4.9749, 12.0104) radius 3.1 projected
  circle A27 centre (0, 0) radius 8 projected
  circle A28 centre (-12.0104, 4.9749) radius 3.1 projected
  circle A29 centre (-4.9749, -12.0104) radius 3.1 projected
  circle A30 centre (12.0104, -4.9749) radius 3.1 projected
  circle A31 centre (4.9749, 12.0104) radius 3.1 projected
  line L15 (28.3615, 44.0022) -> (126.5171, 82.9998)
  arc A32 (126.5171, 82.9998) -> (127.7787, 84.8585) centre (125.7787, 84.8585) ccw
  line L16 (127.7787, 130.9669) -> (127.7787, 84.8585)
  line L17 (127.7787, 130.9669) -> (13, 130.9669)
  line L18 (13, 130.9669) -> (-27.1, 110.9169)
  line L19 (-27.1, 110.9169) -> (-27.1, -31)
  line L20 (-27.1, -31) -> (27.1, -31)
  line L21 (27.1, -31) -> (27.1, 42.1435)
  arc A33 (28.3615, 44.0022) -> (27.1, 42.1435) centre (29.1, 42.1435) ccw
  arc A34 (15, 93.501) -> (13, 95.501) centre (13, 93.501) ccw
  line L22 (15, 93.501) -> (15, 83.501)
  arc A35 (13, 81.501) -> (15, 83.501) centre (13, 83.501) ccw
  line L23 (13, 81.501) -> (-13, 81.501)
  arc A36 (-15, 83.501) -> (-13, 81.501) centre (-13, 83.501) ccw
  line L24 (-15, 83.501) -> (-15, 93.501)
  arc A37 (-13, 95.501) -> (-15, 93.501) centre (-13, 93.501) ccw
  line L25 (-13, 95.501) -> (13, 95.501)
  circle A38 centre (58.8107, 110.101) radius 1.35
  circle A39 centre (112.9107, 100.101) radius 1.75
  circle A40 centre (28.7107, 120.101) radius 1.75
  circle A41 centre (82.8107, 110.101) radius 1.35
  line L26 (51.6203, 95.501) -> (90.0011, 95.501)
  arc A42 (92.0011, 93.501) -> (90.0011, 95.501) centre (90.0011, 93.501) ccw
  line L27 (92.0011, 93.501) -> (92.0011, 83.501)
  arc A43 (90.0011, 81.501) -> (92.0011, 83.501) centre (90.0011, 83.501) ccw
  line L28 (90.0011, 81.501) -> (51.6203, 81.501)
  arc A44 (49.6203, 83.501) -> (51.6203, 81.501) centre (51.6203, 83.501) ccw
  line L29 (49.6203, 83.501) -> (49.6203, 93.501)
  arc A45 (51.6203, 95.501) -> (49.6203, 93.501) centre (51.6203, 93.501) ccw
  circle A46 centre (39.1, 73.501) radius 1.6
  circle A47 centre (70.8107, 122.101) radius 1.35
  circle A48 centre (112.9107, 120.101) radius 1.75
  circle A49 centre (28.7107, 100.101) radius 1.75
  circle A50 centre (49.8107, 73.501) radius 1.6
  circle A51 centre (9.1, 73.501) radius 1.6
  circle A52 centre (-10.9, 73.501) radius 1.6
  circle A53 centre (69.8107, 73.501) radius 1.6
  circle A54 centre (89.8107, 73.501) radius 1.6
  circle A55 centre (12.0104, 1.9749) radius 3.1
  circle A56 centre (4.9749, -15.0104) radius 3.1
  circle A57 centre (-12.0104, -7.9749) radius 3.1
  circle A58 centre (-4.9749, 9.0104) radius 3.1
  circle A59 centre (0, -3) radius 8
  circle A60 centre (-12.0104, 1.9749) radius 3.1
  circle A61 centre (-4.9749, -15.0104) radius 3.1
  circle A62 centre (12.0104, -7.9749) radius 3.1
  circle A63 centre (4.9749, 9.0104) radius 3.1
  line L30 (-13, 86.501) -> (-13, 83.501)
  point P0 (-15, 93.501)
  point P1 (49.6203, 86.501)
  point P2 (-15, 86.501)
  dimension "d167" = 3
  constraints: 32 centre point, 32 end point, 20 point on circle, 1 vertical
  measures "d167" distance of L30.start L30.end
extrude "돌출24" add sketch "스케치22" against normal blind 5 contours L7 A34 L25 A37 L9 A5 L10 A2 | L11 A10 L12 A42 L26 A45 L14 A13
extrude "돌출25" cut sketch "스케치22" against normal blind 5 contours L22 A35 L23 A36 L24 A4 L8 A3 | A12 L13 A11 L27 A43 L28 A44 L29
sketch "스케치23" plane through (0, 5, 0) normal (0, 1, 0) x (1, 0, 0)
  circle A0 centre (4.9749, 12.0104) radius 3.1 projected
  circle A1 centre (12.0104, -4.9749) radius 3.1 projected
  circle A2 centre (-4.9749, -12.0104) radius 3.1 projected
  circle A3 centre (-12.0104, 4.9749) radius 3.1 projected
  circle A4 centre (0, 0) radius 8 projected
  circle A5 centre (-4.9749, 12.0104) radius 3.1 projected
  circle A6 centre (-12.0104, -4.9749) radius 3.1 projected
  circle A7 centre (4.9749, -12.0104) radius 3.1 projected
  circle A8 centre (12.0104, 4.9749) radius 3.1 projected
  circle A9 centre (89.8107, 76.501) radius 1.6 projected
  circle A10 centre (69.8107, 76.501) radius 1.6 projected
  circle A11 centre (-10.9, 76.501) radius 1.6 projected
  circle A12 centre (9.1, 76.501) radius 1.6 projected
  circle A13 centre (49.8107, 76.501) radius 1.6 projected
  circle A14 centre (28.7107, 103.101) radius 1.75 projected
  circle A15 centre (112.9107, 123.101) radius 1.75 projected
  circle A16 centre (70.8107, 125.101) radius 1.35 projected
  circle A17 centre (39.1, 76.501) radius 1.6 projected
  circle A18 centre (82.8107, 113.101) radius 1.35 projected
  circle A19 centre (28.7107, 123.101) radius 1.75 projected
  circle A20 centre (112.9107, 103.101) radius 1.75 projected
  circle A21 centre (58.8107, 113.101) radius 1.35 projected
  line L0 (15, 93.501) -> (15, 83.501) projected
  arc A22 (13, 81.501) -> (15, 83.501) centre (13, 83.501) ccw projected
  line L1 (13, 81.501) -> (-13, 81.501) projected
  arc A23 (-15, 83.501) -> (-13, 81.501) centre (-13, 83.501) ccw projected
  line L2 (-15, 83.501) -> (-15, 93.501) projected
  arc A24 (-13, 95.501) -> (-15, 93.501) centre (-13, 93.501) ccw projected
  line L3 (-13, 95.501) -> (13, 95.501) projected
  arc A25 (15, 93.501) -> (13, 95.501) centre (13, 93.501) ccw projected
  line L4 (28.3615, 47.0022) -> (126.5171, 85.9998) projected
  arc A26 (126.5171, 85.9998) -> (127.7787, 87.8585) centre (125.7787, 87.8585) ccw projected
  line L5 (127.7787, 133.9669) -> (127.7787, 87.8585) projected
  line L6 (127.7787, 133.9669) -> (13, 133.9669) projected
  line L7 (13, 133.9669) -> (-27.1, 113.9169) projected
  line L8 (-27.1, 113.9169) -> (-27.1, -28) projected
  line L9 (-27.1, -28) -> (27.1, -28) projected
  line L10 (27.1, -28) -> (27.1, 45.1435) projected
  arc A27 (28.3615, 47.0022) -> (27.1, 45.1435) centre (29.1, 45.1435) ccw projected
  line L11 (49.6203, 83.501) -> (49.6203, 93.501) projected
  arc A28 (51.6203, 95.501) -> (49.6203, 93.501) centre (51.6203, 93.501) ccw projected
  line L12 (51.6203, 95.501) -> (90.0011, 95.501) projected
  arc A29 (92.0011, 93.501) -> (90.0011, 95.501) centre (90.0011, 93.501) ccw projected
  line L13 (92.0011, 93.501) -> (92.0011, 83.501) projected
  arc A30 (90.0011, 81.501) -> (92.0011, 83.501) centre (90.0011, 83.501) ccw projected
  line L14 (90.0011, 81.501) -> (51.6203, 81.501) projected
  arc A31 (49.6203, 83.501) -> (51.6203, 81.501) centre (51.6203, 83.501) ccw projected
  circle A32 centre (4.9749, 5.0104) radius 3.1
  circle A33 centre (12.0104, -11.9749) radius 3.1
  circle A34 centre (-4.9749, -19.0104) radius 3.1
  circle A35 centre (-12.0104, -2.0251) radius 3.1
  circle A36 centre (0, -7) radius 8
  circle A37 centre (-4.9749, 5.0104) radius 3.1
  circle A38 centre (-12.0104, -11.9749) radius 3.1
  circle A39 centre (4.9749, -19.0104) radius 3.1
  circle A40 centre (12.0104, -2.0251) radius 3.1
  circle A41 centre (89.8107, 69.501) radius 1.6
  circle A42 centre (69.8107, 69.501) radius 1.6
  circle A43 centre (-10.9, 69.501) radius 1.6
  circle A44 centre (9.1, 69.501) radius 1.6
  circle A45 centre (49.8107, 69.501) radius 1.6
  circle A46 centre (28.7107, 96.101) radius 1.75
  circle A47 centre (112.9107, 116.101) radius 1.75
  circle A48 centre (70.8107, 118.101) radius 1.35
  circle A49 centre (39.1, 69.501) radius 1.6
  circle A50 centre (82.8107, 106.101) radius 1.35
  circle A51 centre (28.7107, 116.101) radius 1.75
  circle A52 centre (112.9107, 96.101) radius 1.75
  circle A53 centre (58.8107, 106.101) radius 1.35
  line L15 (15, 86.501) -> (15, 76.501)
  arc A54 (13, 74.501) -> (15, 76.501) centre (13, 76.501) ccw
  line L16 (13, 74.501) -> (-13, 74.501)
  arc A55 (-15, 76.501) -> (-13, 74.501) centre (-13, 76.501) ccw
  line L17 (-15, 76.501) -> (-15, 86.501)
  arc A56 (-13, 88.501) -> (-15, 86.501) centre (-13, 86.501) ccw
  line L18 (-13, 88.501) -> (13, 88.501)
  arc A57 (15, 86.501) -> (13, 88.501) centre (13, 86.501) ccw
  line L19 (28.3615, 40.0022) -> (126.5171, 78.9998)
  arc A58 (126.5171, 78.9998) -> (127.7787, 80.8585) centre (125.7787, 80.8585) ccw
  line L20 (127.7787, 126.9669) -> (127.7787, 80.8585)
  line L21 (127.7787, 126.9669) -> (13, 126.9669)
  line L22 (13, 126.9669) -> (-27.1, 106.9169)
  line L23 (-27.1, 106.9169) -> (-27.1, -35)
  line L24 (-27.1, -35) -> (27.1, -35)
  line L25 (27.1, -35) -> (27.1, 38.1435)
  arc A59 (28.3615, 40.0022) -> (27.1, 38.1435) centre (29.1, 38.1435) ccw
  line L26 (49.6203, 76.501) -> (49.6203, 86.501)
  arc A60 (51.6203, 88.501) -> (49.6203, 86.501) centre (51.6203, 86.501) ccw
  line L27 (51.6203, 88.501) -> (90.0011, 88.501)
  arc A61 (92.0011, 86.501) -> (90.0011, 88.501) centre (90.0011, 86.501) ccw
  line L28 (92.0011, 86.501) -> (92.0011, 76.501)
  arc A62 (90.0011, 74.501) -> (92.0011, 76.501) centre (90.0011, 76.501) ccw
  line L29 (90.0011, 74.501) -> (51.6203, 74.501)
  arc A63 (49.6203, 76.501) -> (51.6203, 74.501) centre (51.6203, 76.501) ccw
  circle A64 centre (70.8107, 125.101) radius 1.35 projected
  line L30 (70.8107, 125.101) -> (70.8107, 118.101)
  point P0 (-27.1, 106.9169)
  dimension "d172" = 7
  constraints: 32 centre point, 32 end point, 20 point on circle, 1 vertical
  measures "d172" distance of L30.start L30.end
extrude "돌출26" add sketch "스케치23" against normal blind 5 contours A14 | A15 | A16 | A18 | A19 | A20 | A21
extrude "돌출27" cut sketch "스케치23" against normal blind 5 contours L21 L22 L8 L7 L6 L5 | A46 | A47 | A48 | A50 | A51 | A52 | A53